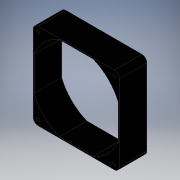
# Autodesk Inventor part: 120mm Fan
Saved by Autodesk Inventor 2016 (Build 200138000, 138)
## iProperties
Created: 2015-10-01
Part Number: 120mm Fan
Material: Generic
Document SubType Name: Modeling
Designer: xdlea
Density: 1 g/cm^3
Appearance: Black
length: 4.685 in
dHoles: 4.126 in
holeSize: 0.177 in
fanDia: 4.921 in
fanCutOff: 4.567 in
Author: xdlea
Autodesk Inventor part; units mm, degrees
ref_plane "YZ Plane" through (0, 0, 0) normal (1, 0, 0) x (0, 1, 0)
ref_plane "XZ Plane" through (0, 0, 0) normal (0, 1, 0) x (-1, 0, 0)
ref_plane "XY Plane" through (0, 0, 0) normal (0, 0, 1) x (1, 0, 0)
sketch "Sketch1" plane through (0, 0, 0) normal (0, 0, 1) x (1, 0, 0)
  line L0 (-59.5, -59.5) -> (59.5, -59.5)
  line L1 (59.5, -59.5) -> (59.5, 59.5)
  line L2 (59.5, 59.5) -> (-59.5, 59.5)
  line L3 (-59.5, 59.5) -> (-59.5, -59.5)
  line L4 (-59.5, -59.5) -> (59.5, 59.5) construction
  line L5 (59.5, -59.5) -> (-59.5, 59.5) construction
  circle A0 centre (-52.4, 52.4) radius 2.25
  circle A1 centre (52.4, 52.4) radius 2.25
  line L6 (-23.2863, -58) -> (23.2863, -58)
  line L7 (58, -23.2863) -> (58, 23.2863)
  line L8 (23.2863, 58) -> (-23.2863, 58)
  line L9 (-58, 23.2863) -> (-58, -23.2863)
  line L10 (-58, -58) -> (58, 58) construction
  line L11 (58, -58) -> (-58, 58) construction
  arc A2 (-58, -23.2863) -> (-23.2863, -58) centre (0, 0) ccw
  arc A3 (23.2863, -58) -> (58, -23.2863) centre (0, 0) ccw
  arc A4 (58, 23.2863) -> (23.2863, 58) centre (0, 0) ccw
  arc A5 (-23.2863, 58) -> (-58, 23.2863) centre (0, 0) ccw
  arc A6 (-52.4, 59.5) -> (-59.5, 52.4) centre (-52.4, 52.4) ccw
  dimension "d0" = 119
  dimension "d2" = 4.5
  dimension "d3" = 104.8
  dimension "d5" = 116
  dimension "d6" = 62.5
  dimension "d7" = 46.5725
  dimension "d15" = 1.5
  constraints: 24 end point, 10 point on circle, 7 centre point, 6 perpendicular, 5 point on line, 4 equal radius, 4 midpoint, 4 parallel, 2 coincident, 2 horizontal, 1 horizontal alignment, 1 tangent
  measures "d0" distance of L2.end L0.start
  measures "d2" diameter of A0
  measures "d3" distance of A1.centre A0.centre
  measures "d5" distance of L10.end L11.end
  measures "d6" radius of A5
  measures "d7" distance of L9.start L9.end
  measures "d15" distance between parallel lines of L3 L9
extrude "Extrusion1" add sketch "Sketch1" along normal blind 38 contours L3 A6 L2 L1 L0 | L3 L2 A6 | A0 | A1
extrude "Extrusion2" cut sketch "Sketch1" along normal blind 38 contours L3 L2 A6 | A0
pattern_circular "Circular Pattern1" count 4 over 360 about axis through (0, 0, 0) along (0, 0, 1) of "Extrusion2"
equation "\"d0\" = length"
equation "\"d2\" = holeSize"
equation "\"d3\" = dHoles"
equation "\"d5\" = fanCutOff"
equation "\"d6\" = 0.5 * fanDia"
equation "\"d8\" = heigth"
equation "\"d10\" = heigth"
equation "\"length\" = 119"
equation "\"width\" = length"
equation "\"heigth\" = 38"
equation "\"dHoles\" = 104.8"
equation "\"holeSize\" = 4.5"
equation "\"fanDia\" = 125"
equation "\"fanCutOff\" = 116"
equation "\"d4\" = fanDia"
body "Solid1"
